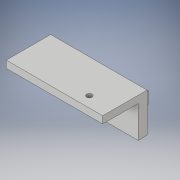
# Autodesk Inventor part: КВ33.044.703 - Стойка оптического датчика оси Y
Saved by Autodesk Inventor 2019 (Build 230136000, 136)
## iProperties
Created: 2019-08-26
Part Number: КВ33.044.703 - Стойка оптического датчика оси Y
Material: Типовые
Document SubType Name: Modeling
Designer: Петров Иван
Density: 1 g/cm^3
Appearance: По умолчанию
Author: Петров Иван
Autodesk Inventor part; units mm, degrees
ref_plane "YZ Plane" through (0, 0, 0) normal (1, 0, 0) x (0, 1, 0)
ref_plane "XZ Plane" through (0, 0, 0) normal (0, 1, 0) x (-1, 0, 0)
ref_plane "XY Plane" through (0, 0, 0) normal (0, 0, 1) x (1, 0, 0)
sketch "Эскиз1" plane through (0, 0, 0) normal (0, 1, 0) x (-1, 0, 0)
  circle A0 centre (24.25, -12.5) radius 1.95
  circle A1 centre (44.25, -12.5) radius 1.95
  line L0 (68.5, 0) -> (0, 0)
  line L1 (0, 0) -> (0, -5)
  line L2 (14.449, -5) -> (0, -5)
  line L3 (14.449, -5) -> (14.449, -20)
  line L4 (14.449, -20) -> (54.25, -20)
  line L5 (54.25, -5) -> (54.25, -20)
  line L6 (68.5, -5) -> (54.25, -5)
  line L7 (68.5, 0) -> (68.5, -5)
  point P0 (-5.75, 0)
  constraints: 16 end point, 2 centre point
extrude "Выдавливание1" add sketch "Эскиз1" along normal blind 22
sketch "Эскиз2" plane through (-68.5, 0, 0) normal (0, 0, 1) x (1, 0, 0)
  line L0 (0, 0) -> (0, 22) projected
  line L1 (0, 22) -> (68.5, 22) projected
  line L2 (68.5, 0) -> (68.5, 22) projected
  line L3 (0, 22) -> (68.5, 22)
  line L4 (68.5, 22) -> (68.5, 18)
  line L5 (68.5, 18) -> (0, 18)
  line L6 (0, 18) -> (0, 22)
  dimension "d2" = 4
  constraints: 8 end point, 2 parallel, 1 horizontal, 1 perpendicular, 1 point on line
  measures "d2" distance of L3.end L4.end
extrude "Выдавливание2" add sketch "Эскиз2" along normal blind 20
sketch "Эскиз3" plane through (0, 22, 0) normal (0, 1, 0) x (1, 0, 0)
  line L0 (0, 5) -> (-14.449, 5) projected
  line L1 (-54.25, 20) -> (-14.449, 20)
  line L2 (-14.449, 20) -> (-14.449, 5)
  line L3 (-14.449, 5) -> (-54.25, 5)
  line L4 (-54.25, 5) -> (-54.25, 20)
  point P0 (0, 0)
  constraints: 8 end point, 2 parallel, 1 horizontal, 1 perpendicular
extrude "Выдавливание3" cut sketch "Эскиз3" against normal blind 15
sketch "Эскиз4" plane through (0, 22, 0) normal (0, 1, 0) x (1, 0, 0)
  line L0 (-68.5, -20) -> (0, -20) projected
  line L1 (0, -20) -> (-13.5, -20)
  line L2 (-13.5, -20) -> (-13.5, -14)
  line L3 (-13.5, -14) -> (0, -14)
  line L4 (0, -14) -> (0, -20)
  circle A0 centre (-13.5, -14) radius 1.5
  point P0 (0, 0)
  dimension "d7" = 13.5
  dimension "d8" = 6
  dimension "d9" = 3
  constraints: 8 end point, 2 parallel, 1 centre point, 1 coincident, 1 horizontal, 1 perpendicular
  measures "d7" distance of L2.end L3.end
  measures "d8" distance of L1.end L2.end
  measures "d9" diameter of A0
extrude "Выдавливание4" cut sketch "Эскиз4" against normal blind 15 contours A0 L3 L2 | L2 L3 A0
move faces "Перенос1" translate (14.25, 0, 0) faces at (-68.5, 13.3333, -3.3333)
